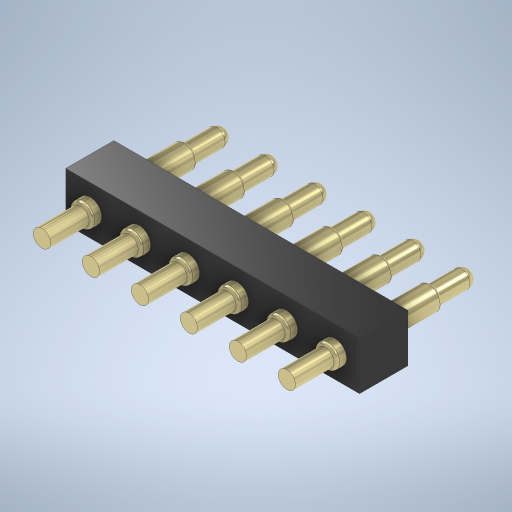
# Autodesk Inventor part: PogoPins - 1x6Array
Saved by Autodesk Inventor 2023 (Build 270158000, 158)
## iProperties
Created: 2023-01-23
Part Number: PogoPins - 1x6Array
Material: Generic
Document SubType Name: Modeling
Designer: Administrator
Density: 1 g/cm^3
Appearance: Default
Author: Administrator
Autodesk Inventor part; units mm, degrees
ref_plane "YZ Plane" through (0, 0, 0) normal (1, 0, 0) x (0, 1, 0)
ref_plane "XZ Plane" through (0, 0, 0) normal (0, 1, 0) x (-1, 0, 0)
ref_plane "XY Plane" through (0, 0, 0) normal (0, 0, 1) x (1, 0, 0)
sketch "Sketch1" plane through (0, 0, 0) normal (0, 0, 1) x (1, 0, 0)
  circle A0 centre (0, 0) radius 0.6
  circle A1 centre (2.54, 0) radius 0.6
  circle A2 centre (5.08, 0) radius 0.6
  circle A3 centre (7.62, 0) radius 0.6
  circle A4 centre (10.16, 0) radius 0.6
  circle A5 centre (12.7, 0) radius 0.6
  line L0 (-1.27, 1.25) -> (13.97, 1.25)
  line L1 (13.97, 1.25) -> (13.97, -1.25)
  line L2 (13.97, -1.25) -> (-1.27, -1.25)
  line L3 (-1.27, -1.25) -> (-1.27, 1.25)
  line L4 (0, 0) -> (12.7, 0) construction
  point P0 (13.97, 0)
  dimension "d0" = 1.2
  dimension "d1" = 1.2
  dimension "d2" = 1.2
  dimension "d3" = 1.2
  dimension "d4" = 1.2
  dimension "d5" = 1.2
  dimension "d6" = 2.54
  dimension "d7" = 2.54
  dimension "d8" = 2.54
  dimension "d9" = 2.54
  dimension "d10" = 2.54
  dimension "d11" = 2.5
  dimension "d12" = 1.27
  dimension "d13" = 1.27
  dimension "d14" = 0
  constraints: 10 end point, 6 centre point, 4 point on line, 2 horizontal, 2 parallel, 1 coincident, 1 midpoint, 1 perpendicular
  measures "d0" diameter of A0
  measures "d1" diameter of A1
  measures "d2" diameter of A2
  measures "d3" diameter of A3
  measures "d4" diameter of A4
  measures "d5" diameter of A5
  measures "d6" distance of A1.centre point (0, 0)
  measures "d7" distance of A2.centre A1.centre
  measures "d8" distance of A3.centre A2.centre
  measures "d9" distance of A3.centre A4.centre
  measures "d10" distance of A4.centre L4.end
  measures "d11" distance of L0.end L1.end
  measures "d12" distance from line of L3 point (0, 0)
  measures "d13" distance of point (13.97, 0) L4.end
  measures "d14" vertical distance of point (13.97, 0) L4.end
extrude "Extrusion1" add sketch "Sketch1" along normal mid plane 2.5 contours A0 | A1 | A2 | A3 | A4 | A5 | L0 L1 L2 L3
extrude "Extrusion2" add sketch "Sketch1" along normal blind 1.75 contours A0 | A1 | A2 | A3 | A4 | A5
extrude "Extrusion3" add sketch "Sketch1" against normal blind 3.75 contours A0 | A1 | A2 | A3 | A4 | A5
sketch "Sketch2" plane through (0, 0, 1.75) normal (0, 0, 1) x (1, 0, 0)
  circle A0 centre (0, 0) radius 0.6 projected
  circle A1 centre (2.54, 0) radius 0.6 projected
  circle A2 centre (5.08, 0) radius 0.6 projected
  circle A3 centre (7.62, 0) radius 0.6 projected
  circle A4 centre (10.16, 0) radius 0.6 projected
  circle A5 centre (12.7, 0) radius 0.6 projected
  circle A6 centre (0, 0) radius 0.45
  line L0 (0, 0) -> (12.7, 0) construction
  circle A7 centre (2.54, 0) radius 0.45
  circle A8 centre (5.08, 0) radius 0.45
  circle A9 centre (7.62, 0) radius 0.45
  circle A10 centre (10.16, 0) radius 0.45
  circle A11 centre (12.7, 0) radius 0.45
  dimension "d21" = 0.9
  dimension "d24" = 2.54
  constraints: 6 centre point, 2 end point, 2 horizontal, 1 coincident, 10 other
  measures "d21" diameter of A6
  measures "d24" distance of L0.start A7.centre
extrude "Extrusion4" add sketch "Sketch2" along normal blind 2 and the other way blind 7.5 contours A6 | A7 | A8 | A9 | A10 | A11
fillet "Fillet1" radius 0.15 12 edges at (-0.6, 0, 1.75) (1.94, 0, 1.75) (4.48, 0, 1.75) (7.02, 0, 1.75) (9.56, 0, 1.75) (12.1, 0, 1.75) (12.1, 0, -3.75) (9.56, 0, -3.75) (7.02, 0, -3.75) (4.48, 0, -3.75) (1.94, 0, -3.75) (-0.6, 0, -3.75)
fillet "Fillet2" radius 0.45 6 edges at (12.25, 0, -5.75) (9.71, 0, -5.75) (7.17, 0, -5.75) (4.63, 0, -5.75) (2.09, 0, -5.75) (-0.45, 0, -5.75)
equation "\"d7\" = d6"
equation "\"d8\" = d6"
equation "\"d9\" = d6"
equation "\"d10\" = d6"
equation "\"d12\" = 0.5 * d6"
equation "\"d13\" = 0.5 * d6"
body "Solid1"
